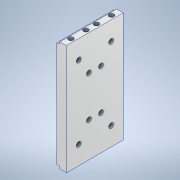
# Autodesk Inventor part: Vertical Vìnculo Cabezal
Saved by Autodesk Inventor 2020 (Build 240168000, 168)
## iProperties
Created: 2020-05-16
Part Number: Vertical Vìnculo Cabezal
Material: Aluminum 6061
Document SubType Name: Modeling
Designer: Dante
Density: 2.7 g/cm^3
Appearance: Aluminum - Flat
Mass: 285.251 g
Surface Area: 282.104 cm^2
Volume: 105.649 cm^3
Author: Dante
Autodesk Inventor part; units mm, degrees
ref_plane "YZ Plane" through (0, 0, 0) normal (1, 0, 0) x (0, 1, 0)
ref_plane "XZ Plane" through (0, 0, 0) normal (0, 1, 0) x (-1, 0, 0)
ref_plane "XY Plane" through (0, 0, 0) normal (0, 0, 1) x (1, 0, 0)
sketch "Sketch1" plane through (0, 0, 0) normal (0, 0, 1) x (1, 0, 0)
  line L0 (0.0233, 9.5241) -> (9.0233, 9.5241)
  line L1 (0.0233, 9.5241) -> (0.0233, 6.5241)
  line L2 (0.0233, 6.5241) -> (-2.9767, 6.5241)
  line L3 (-2.9767, 6.5241) -> (-2.9767, -123.4759)
  line L4 (-2.9767, -123.4759) -> (0.0233, -123.4759)
  line L5 (0.0233, -123.4759) -> (0.0233, -126.4759)
  line L6 (0.0233, -126.4759) -> (9.0233, -126.4759)
  line L7 (9.0233, -126.4759) -> (9.0233, 9.5241)
  dimension "d0" = 9
  dimension "d1" = 3
  dimension "d2" = 3
  dimension "d3" = 130
  dimension "d4" = 3
  dimension "d5" = 9
  constraints: 16 end point, 5 perpendicular, 2 vertical, 1 horizontal
  measures "d0" distance of L0.start L0.end
  measures "d1" distance of L0.start L1.end
  measures "d2" distance of L1.end L2.end
  measures "d3" distance of L2.end L3.end
  measures "d4" distance of L4.end L5.end
  measures "d5" distance of L5.end L6.end
extrude "Extrusion1" add sketch "Sketch1" along normal blind 70
sketch "Sketch2" plane through (0.0233, 9.5241, 0) normal (0, 1, 0) x (1, 0, 0)
  circle A0 centre (4.5, -10) radius 3
  circle A1 centre (4.5, -28.5) radius 3
  circle A2 centre (4.5, -41.5) radius 3
  circle A3 centre (4.5, -60) radius 3
  line L0 (9, -70) -> (0, -70) projected
  line L1 (9, 0) -> (0, 0) projected
  line L2 (0, 0) -> (0, -70) projected
  point P0 (-0.0233, 0)
  dimension "d8" = 6
  dimension "d9" = 6
  dimension "d10" = 6
  dimension "d11" = 6
  dimension "d12" = 10
  dimension "d16" = 10
  dimension "d18" = 4.5
  dimension "d19" = 4.5
  dimension "d20" = 4.5
  dimension "d21" = 4.5
  dimension "d135" = 28.5
  dimension "d136" = 28.5
  constraints: 4 centre point
  measures "d8" diameter of A0
  measures "d9" diameter of A1
  measures "d10" diameter of A2
  measures "d11" diameter of A3
  measures "d12" distance from line of L0 A3.centre
  measures "d16" distance from line of L1 A0.centre
  measures "d18" distance from line of L2 A0.centre
  measures "d19" distance from line of L2 A1.centre
  measures "d20" distance from line of L2 A2.centre
  measures "d21" distance from line of L2 A3.centre
  measures "d135" distance from line of A1.centre L1
  measures "d136" distance from line of L0 A2.centre
sketch "Sketch3" plane through (0.0233, -126.4759, 0) normal (0, -1, 0) x (1, 0, 0)
  circle A0 centre (4.5, 10) radius 3
  circle A1 centre (4.5, 28.5) radius 3
  circle A2 centre (4.5, 41.5) radius 3
  circle A3 centre (4.5, 60) radius 3
  line L0 (0, 70) -> (9, 70) projected
  line L1 (0, 0) -> (9, 0) projected
  line L2 (0, 0) -> (0, 70) projected
  point P0 (-0.0233, 0)
  dimension "d38" = 6
  dimension "d39" = 6
  dimension "d40" = 6
  dimension "d41" = 6
  dimension "d42" = 10
  dimension "d43" = 10
  dimension "d46" = 4.5
  dimension "d47" = 4.5
  dimension "d48" = 4.5
  dimension "d49" = 4.5
  dimension "d137" = 28.5
  dimension "d138" = 28.5
  constraints: 4 centre point
  measures "d38" diameter of A0
  measures "d39" diameter of A1
  measures "d40" diameter of A2
  measures "d41" diameter of A3
  measures "d42" distance from line of L0 A3.centre
  measures "d43" distance from line of L1 A0.centre
  measures "d46" distance from line of L2 A2.centre
  measures "d47" distance from line of L2 A3.centre
  measures "d48" distance from line of L2 A1.centre
  measures "d49" distance from line of L2 A0.centre
  measures "d137" distance from line of L1 A1.centre
  measures "d138" distance from line of L0 A2.centre
sketch "Sketch4" plane through (-2.9767, -123.4759, 0) normal (-1, 0, 0) x (0, 0, 1)
  circle A0 centre (15, 110) radius 3
  circle A1 centre (27.5, 90) radius 3
  circle A2 centre (42.5, 90) radius 3
  circle A3 centre (55, 110) radius 3
  line L0 (0, 133) -> (70, 133) projected
  line L1 (0, 130) -> (0, 0) projected
  line L2 (70, 130) -> (70, 0) projected
  line L3 (70, -3) -> (70, 133) projected
  line L4 (70, 65) -> (60.0222, 65)
  circle A4 centre (15, 20) radius 3
  circle A5 centre (27.5, 40) radius 3
  circle A6 centre (42.5, 40) radius 3
  circle A7 centre (55, 20) radius 3
  circle A8 centre (15, 110) radius 5.125
  circle A9 centre (27.5, 90) radius 5.125
  circle A10 centre (42.5, 90) radius 5.125
  circle A11 centre (55, 110) radius 5.125
  circle A12 centre (15, 20) radius 5.125
  circle A13 centre (27.5, 40) radius 5.125
  circle A14 centre (42.5, 40) radius 5.125
  circle A15 centre (55, 20) radius 5.125
  circle A16 centre (35, 65) radius 3
  line L5 (35, 65) -> (35, 82.0143)
  circle A17 centre (60, 82.0143) radius 3
  circle A18 centre (45, 82.0143) radius 3
  circle A19 centre (10, 86.2004) radius 3
  point P0 (0, 123.4759)
  dimension "d52" = 6
  dimension "d53" = 6
  dimension "d54" = 6
  dimension "d55" = 6
  dimension "d56" = 23
  dimension "d57" = 43
  dimension "d58" = 43
  dimension "d59" = 23
  dimension "d60" = 15
  dimension "d61" = 15
  dimension "d66" = 10.25
  dimension "d67" = 10.25
  dimension "d68" = 10.25
  dimension "d69" = 10.25
  dimension "d70" = 10.25
  dimension "d71" = 10.25
  dimension "d72" = 10.25
  dimension "d73" = 10.25
  dimension "d76" = 6
  dimension "d77" = 6
  dimension "d78" = 6
  dimension "d79" = 10
  dimension "d80" = 15
  dimension "d83" = 6
  dimension "d85" = 10
  dimension "d133" = 12.5
  dimension "d134" = 12.5
  constraints: 20 centre point, 8 coincident, 4 end point, 4 symmetric about line, 1 horizontal, 1 midpoint, 1 point on line, 1 vertical, 4 other
  measures "d52" diameter of A0
  measures "d53" diameter of A1
  measures "d54" diameter of A2
  measures "d55" diameter of A3
  measures "d56" distance from line of L0 A0.centre
  measures "d57" distance from line of L0 A1.centre
  measures "d58" distance from line of L0 A2.centre
  measures "d59" distance from line of L0 A3.centre
  measures "d60" distance from line of L1 A0.centre
  measures "d61" distance from line of A3.centre L2
  measures "d66" diameter of A8
  measures "d67" diameter of A9
  measures "d68" diameter of A10
  measures "d69" diameter of A11
  measures "d70" diameter of A12
  measures "d71" diameter of A13
  measures "d72" diameter of A14
  measures "d73" diameter of A15
  measures "d76" diameter of A16
  measures "d77" diameter of A17
  measures "d78" diameter of A18
  measures "d79" distance from line of A17.centre L2
  measures "d80" distance of A18.centre A17.centre
  measures "d83" diameter of A19
  measures "d85" distance from line of L1 A19.centre
  measures "d133" horizontal distance of A2.centre A3.centre
  measures "d134" horizontal distance of A0.centre A1.centre
extrude "Extrusion5" cut sketch "Sketch4" against normal blind 21 contours A0 | A1 | A2 | A3 | A4 | A5 | A6 | A7
hole "Agujero1" at (4.5233, 9.5241, 10) at (4.5233, 9.5241, 28.5) at (4.5233, 9.5241, 41.5) at (4.5233, 9.5241, 60) direction (0, -1, 0) diameter 6 depth 15 tip angle 118
hole "Agujero2" at (4.5233, -126.4759, 10) at (4.5233, -126.4759, 28.5) at (4.5233, -126.4759, 41.5) at (4.5233, -126.4759, 60) direction (0, 1, 0) diameter 6 depth 15 tip angle 118
thread "Rosca9" size "M6x1" class "6H" standard "ISO Metric profile" length 10
thread "Rosca10" size "M6x1" class "6H" standard "ISO Metric profile" length 10
thread "Rosca11" size "M6x1" class "6H" standard "ISO Metric profile" length 10
thread "Rosca12" size "M6x1" class "6H" standard "ISO Metric profile" length 10
thread "Rosca13" size "M6x1" class "6H" standard "ISO Metric profile" length 10
thread "Rosca14" size "M6x1" class "6H" standard "ISO Metric profile" length 10
thread "Rosca15" size "M6x1" class "6H" standard "ISO Metric profile" length 10
thread "Rosca16" size "M6x1" class "6H" standard "ISO Metric profile" length 10
chamfer "Chaflán1" distance 1 angle 45 2 edges at (0.0233, 9.5241, 35) (0.0233, -126.4759, 35)
equation "\"d16\" = d12"
equation "\"d136\" = d135"
equation "\"d43\" = d42"
equation "\"d138\" = d137"
body "Solid1"
